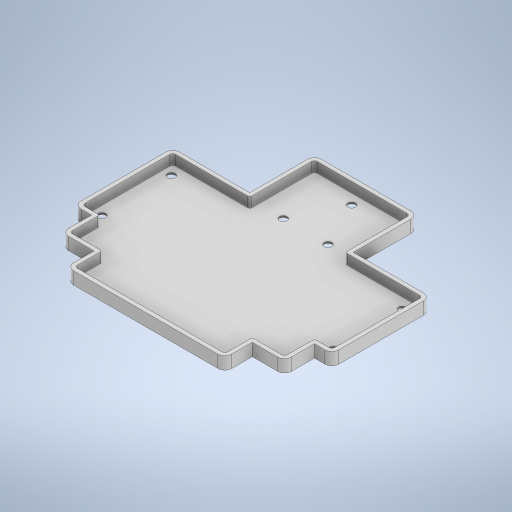
# Autodesk Inventor part: forma_podstawa
Saved by Autodesk Inventor 2023 (Build 270158000, 158)
## iProperties
Created: 2025-03-20
Part Number: forma_podstawa
Material: Ogólny
Document SubType Name: Modeling
Designer: kamil
Density: 1 g/cm^3
Appearance: Domyślna
Author: kamil
Autodesk Inventor part; units mm, degrees
ref_plane "YZ Plane" through (0, 0, 0) normal (1, 0, 0) x (0, 1, 0)
ref_plane "XZ Plane" through (0, 0, 0) normal (0, 1, 0) x (-1, 0, 0)
ref_plane "XY Plane" through (0, 0, 0) normal (0, 0, 1) x (1, 0, 0)
sketch "Szkic1" plane through (0, 0, 0) normal (0, 1, 0) x (-1, 0, 0)
  arc A0 (49, -17.5404) -> (50, -16.5404) centre (49, -16.5404) ccw
  line L0 (20, -17.5404) -> (49, -17.5404)
  line L1 (50, -16.5404) -> (50, 17.4596)
  arc A1 (50, 17.4596) -> (49, 18.4596) centre (49, 17.4596) ccw
  line L2 (49, 18.4596) -> (44, 18.4596)
  arc A2 (43, 19.4596) -> (44, 18.4596) centre (44, 19.4596) ccw
  line L3 (43, 19.4596) -> (43, 29.4596)
  line L4 (42, 30.4596) -> (31, 30.4596)
  arc A3 (43, 29.4596) -> (42, 30.4596) centre (42, 29.4596) ccw
  arc A4 (30, 31.4596) -> (31, 30.4596) centre (31, 31.4596) ccw
  line L5 (30, 31.4596) -> (30, 40.4596)
  arc A5 (30, 40.4596) -> (29, 41.4596) centre (29, 40.4596) ccw
  line L6 (29, 41.4596) -> (-29, 41.4596)
  line L7 (-30, 40.4596) -> (-30, 31.4596)
  arc A6 (-29, 41.4596) -> (-30, 40.4596) centre (-29, 40.4596) ccw
  arc A7 (-31, 30.4596) -> (-30, 31.4596) centre (-31, 31.4596) ccw
  line L8 (-31, 30.4596) -> (-42, 30.4596)
  arc A8 (-42, 30.4596) -> (-43, 29.4596) centre (-42, 29.4596) ccw
  line L9 (-43, 29.4596) -> (-43, 19.4596)
  arc A9 (-44, 18.4596) -> (-43, 19.4596) centre (-44, 19.4596) ccw
  line L10 (-44, 18.4596) -> (-49, 18.4596)
  arc A10 (-49, 18.4596) -> (-50, 17.4596) centre (-49, 17.4596) ccw
  line L11 (-50, 17.4596) -> (-50, -16.5404)
  line L12 (-49, -17.5404) -> (-20, -17.5404)
  arc A11 (-50, -16.5404) -> (-49, -17.5404) centre (-49, -16.5404) ccw
  arc A12 (-19, -18.5404) -> (-20, -17.5404) centre (-20, -18.5404) ccw
  line L13 (-19, -18.5404) -> (-19, -42.5404)
  arc A13 (20, -17.5404) -> (19, -18.5404) centre (20, -18.5404) ccw
  line L14 (19, -42.5404) -> (19, -18.5404)
  line L15 (-18, -43.5404) -> (18, -43.5404)
  arc A14 (18, -43.5404) -> (19, -42.5404) centre (18, -42.5404) ccw
  arc A15 (-19, -42.5404) -> (-18, -43.5404) centre (-18, -42.5404) ccw
  circle A16 centre (0, -39.5) radius 1.5
  circle A17 centre (9, -21) radius 1.5
  circle A18 centre (-9, -21) radius 1.5
  circle A19 centre (-46.5, -13.5) radius 1.5
  circle A20 centre (46.5, -13.5) radius 1.5
  circle A21 centre (46.5, 14.3844) radius 1.5
  circle A22 centre (-46.5, 14.3844) radius 1.5
  arc A23 (49, -17.7404) -> (50.2, -16.5404) centre (49, -16.5404) ccw
  line L16 (50.2, -16.5404) -> (50.2, 17.4596)
  arc A24 (50.2, 17.4596) -> (49, 18.6596) centre (49, 17.4596) ccw
  line L17 (49, 18.6596) -> (44, 18.6596)
  arc A25 (43.2, 19.4596) -> (44, 18.6596) centre (44, 19.4596) ccw
  line L18 (43.2, 19.4596) -> (43.2, 29.4596)
  arc A26 (43.2, 29.4596) -> (42, 30.6596) centre (42, 29.4596) ccw
  line L19 (42, 30.6596) -> (31, 30.6596)
  arc A27 (30.2, 31.4596) -> (31, 30.6596) centre (31, 31.4596) ccw
  line L20 (30.2, 31.4596) -> (30.2, 40.4596)
  arc A28 (30.2, 40.4596) -> (29, 41.6596) centre (29, 40.4596) ccw
  line L21 (29, 41.6596) -> (-29, 41.6596)
  arc A29 (-29, 41.6596) -> (-30.2, 40.4596) centre (-29, 40.4596) ccw
  line L22 (-30.2, 40.4596) -> (-30.2, 31.4596)
  arc A30 (-31, 30.6596) -> (-30.2, 31.4596) centre (-31, 31.4596) ccw
  line L23 (-31, 30.6596) -> (-42, 30.6596)
  arc A31 (-42, 30.6596) -> (-43.2, 29.4596) centre (-42, 29.4596) ccw
  line L24 (-43.2, 29.4596) -> (-43.2, 19.4596)
  arc A32 (-44, 18.6596) -> (-43.2, 19.4596) centre (-44, 19.4596) ccw
  line L25 (-44, 18.6596) -> (-49, 18.6596)
  arc A33 (-49, 18.6596) -> (-50.2, 17.4596) centre (-49, 17.4596) ccw
  line L26 (-50.2, 17.4596) -> (-50.2, -16.5404)
  arc A34 (-50.2, -16.5404) -> (-49, -17.7404) centre (-49, -16.5404) ccw
  line L27 (-49, -17.7404) -> (-20, -17.7404)
  arc A35 (-19.2, -18.5404) -> (-20, -17.7404) centre (-20, -18.5404) ccw
  line L28 (-19.2, -18.5404) -> (-19.2, -42.5404)
  arc A36 (-19.2, -42.5404) -> (-18, -43.7404) centre (-18, -42.5404) ccw
  line L29 (-18, -43.7404) -> (18, -43.7404)
  arc A37 (18, -43.7404) -> (19.2, -42.5404) centre (18, -42.5404) ccw
  line L30 (19.2, -42.5404) -> (19.2, -18.5404)
  arc A38 (20, -17.7404) -> (19.2, -18.5404) centre (20, -18.5404) ccw
  line L31 (20, -17.7404) -> (49, -17.7404)
  arc A39 (49, -19.3404) -> (51.8, -16.5404) centre (49, -16.5404) ccw
  line L32 (51.8, -16.5404) -> (51.8, 17.4596)
  arc A40 (51.8, 17.4596) -> (49, 20.2596) centre (49, 17.4596) ccw
  line L33 (49, 20.2596) -> (44.8, 20.2596)
  line L34 (44.8, 20.2596) -> (44.8, 29.4596)
  arc A41 (44.8, 29.4596) -> (42, 32.2596) centre (42, 29.4596) ccw
  line L35 (42, 32.2596) -> (31.8, 32.2596)
  line L36 (31.8, 32.2596) -> (31.8, 40.4596)
  arc A42 (31.8, 40.4596) -> (29, 43.2596) centre (29, 40.4596) ccw
  line L37 (29, 43.2596) -> (-29, 43.2596)
  arc A43 (-29, 43.2596) -> (-31.8, 40.4596) centre (-29, 40.4596) ccw
  line L38 (-31.8, 40.4596) -> (-31.8, 32.2596)
  line L39 (-31.8, 32.2596) -> (-42, 32.2596)
  arc A44 (-42, 32.2596) -> (-44.8, 29.4596) centre (-42, 29.4596) ccw
  line L40 (-44.8, 29.4596) -> (-44.8, 20.2596)
  line L41 (-44.8, 20.2596) -> (-49, 20.2596)
  arc A45 (-49, 20.2596) -> (-51.8, 17.4596) centre (-49, 17.4596) ccw
  line L42 (-51.8, 17.4596) -> (-51.8, -16.5404)
  arc A46 (-51.8, -16.5404) -> (-49, -19.3404) centre (-49, -16.5404) ccw
  line L43 (-49, -19.3404) -> (-20.8, -19.3404)
  line L44 (-20.8, -19.3404) -> (-20.8, -42.5404)
  arc A47 (-20.8, -42.5404) -> (-18, -45.3404) centre (-18, -42.5404) ccw
  line L45 (-18, -45.3404) -> (18, -45.3404)
  arc A48 (18, -45.3404) -> (20.8, -42.5404) centre (18, -42.5404) ccw
  line L46 (20.8, -42.5404) -> (20.8, -19.3404)
  line L47 (20.8, -19.3404) -> (49, -19.3404)
  point P0 (0, 0)
  point P1 (0, 0)
  dimension "d0" = 0.2
  dimension "d1" = 1.6
  constraints: 96 end point, 84 point on circle, 49 centre point, 56 other
  measures "d0" distance between parallel lines of L0 L31
  measures "d1" distance between parallel lines of L31 L47
extrude "Wyciągnięcie proste1" add sketch "Szkic1" along normal blind 1 contours L0 A13 L14 A14 L15 A15 L13 A12 L12 A11 L11 A10 L10 A9 L9 A8 L8 A7 L7 A6 L6 A5 L5 A4 L4 A3 L3 A2 L2 A1 L1 A0 | L31 A38 L30 A37 L29 A36 L28 A35 L27 A34 L26 A33 L25 A32 L24 A31 L23 A30 L22 A29 L21 A28 L20 A27 L19 A26 L18 A25 L17 A24 L16 A23 | L47 L46 A48 L45 A47 L44 L43 A46 L42 A45 L41 L40 A44 L39 L38 A43 L37 A42 L36 L35 A41 L34 L33 A40 L32 A39
extrude "Wyciągnięcie proste2" add sketch "Szkic1" along normal blind 5 contours L47 L46 A48 L45 A47 L44 L43 A46 L42 A45 L41 L40 A44 L39 L38 A43 L37 A42 L36 L35 A41 L34 L33 A40 L32 A39
fillet "Zaokrąglenie1" radius 0.6 7 edges at (48, 0, -13.5) (10.5, 0, -21) (1.5, 0, -39.5) (-7.5, 0, -21) (48, 0, 14.3844) (-45, 0, 14.3844) (-45, 0, -13.5)
